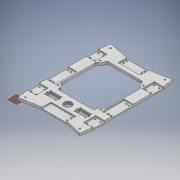
# Autodesk Inventor part: 3枚目
Saved by Autodesk Inventor 2018 (Build 220112000, 112)
## iProperties
Created: 2018-08-16
Part Number: 3枚目
Material: 一般
Document SubType Name: Modeling
Designer: shun2
Density: 1 g/cm^3
Appearance: 既定
Author: shun2
Autodesk Inventor part; units mm, degrees
ref_plane "YZ Plane" through (0, 0, 0) normal (1, 0, 0) x (0, 1, 0)
ref_plane "XZ Plane" through (0, 0, 0) normal (0, 1, 0) x (-1, 0, 0)
ref_plane "XY Plane" through (0, 0, 0) normal (0, 0, 1) x (1, 0, 0)
ref_plane "作業平面1" through (0, 0, 5.5) normal (0, 0, 1) x (1, 0, 0)
sketch "スケッチ3" plane through (0, 0, 5.5) normal (0, 0, 1) x (1, 0, 0)
  line L0 (0, 171.7239) -> (0, 23)
  line L1 (0, 23) -> (3, 0)
  line L2 (136, 23) -> (136, 171.7239)
  line L3 (136, 171.7239) -> (133.0079, 194.6636)
  line L4 (0, 23) -> (0, 75)
  line L5 (0, 127.7239) -> (0, 171.7239)
  line L6 (136, 171.7239) -> (136, 119.7239)
  line L7 (136, 67) -> (136, 23)
  circle A0 centre (11, 186.7239) radius 1.6
  circle A1 centre (125, 186.7239) radius 1.6
  circle A2 centre (11, 8) radius 1.6
  circle A3 centre (125, 8) radius 1.6
  line L8 (6.4, 186.7239) -> (15.6, 186.7239)
  line L9 (11, 182.1239) -> (11, 191.3239)
  line L10 (120.4, 186.7239) -> (129.6, 186.7239)
  line L11 (125, 182.1239) -> (125, 191.3239)
  line L12 (6.4, 8) -> (15.6, 8)
  line L13 (11, 3.4) -> (11, 12.6)
  line L14 (120.4, 8) -> (129.6, 8)
  line L15 (0, 127.7239) -> (0, 171.7239)
  line L16 (136, 171.7239) -> (136, 119.7239)
  line L17 (136, 67) -> (136, 23)
  line L18 (0, 23) -> (0, 75)
  line L19 (133, 0) -> (136, 23)
  line L20 (136, 46) -> (136, 23)
  line L21 (136, 23) -> (117.7, 23)
  line L22 (117.7, 23) -> (117.7, 48.5)
  line L23 (117.7, 48.5) -> (136, 48.5)
  line L24 (136, 48.5) -> (136, 23)
  line L25 (0, 23) -> (18.3, 23)
  line L26 (18.3, 23) -> (18.3, 48.5)
  line L27 (18.3, 48.5) -> (0, 48.5)
  line L28 (0, 48.5) -> (0, 23)
  line L29 (136, 171.7239) -> (117.7, 171.7239)
  line L30 (117.7, 171.7239) -> (117.7, 146.2239)
  line L31 (117.7, 146.2239) -> (136, 146.2239)
  line L32 (136, 146.2239) -> (136, 171.7239)
  line L33 (0, 171.7239) -> (18.3, 171.7239)
  line L34 (18.3, 171.7239) -> (18.3, 146.2239)
  line L35 (18.3, 146.2239) -> (0, 146.2239)
  line L36 (0, 146.2239) -> (0, 171.7239)
  circle A4 centre (132, 27) radius 1.6
  circle A5 centre (121.2, 27) radius 1.6
  circle A6 centre (132, 44.5) radius 1.6
  circle A7 centre (121.2, 44.5) radius 1.6
  circle A8 centre (132, 150.2239) radius 1.6
  circle A9 centre (132, 167.7239) radius 1.6
  circle A10 centre (121.2, 150.2239) radius 1.6
  circle A11 centre (121.2, 167.7239) radius 1.6
  circle A12 centre (14.8, 27) radius 1.6
  circle A13 centre (4, 27) radius 1.6
  circle A14 centre (14.8, 44.5) radius 1.6
  circle A15 centre (4, 44.5) radius 1.6
  circle A16 centre (14.8, 150.2239) radius 1.6
  circle A17 centre (4, 150.2239) radius 1.6
  circle A18 centre (14.8, 167.7239) radius 1.6
  circle A19 centre (4, 167.7239) radius 1.6
  line L37 (98, 8) -> (133, 0)
  line L38 (46.1667, 8) -> (3, 0)
  line L39 (98, 8) -> (46.1667, 8)
  line L40 (46.1667, 8) -> (46.1667, 26.3)
  line L41 (46.1667, 26.3) -> (98, 26.3)
  line L42 (98, 26.3) -> (98, 8)
  circle A20 centre (94, 12.65) radius 1.6
  circle A21 centre (94, 21.65) radius 1.6
  line L43 (68, 186.7239) -> (90.813, 186.7239)
  line L44 (90.813, 186.7239) -> (90.813, 168.4239)
  line L45 (90.813, 168.4239) -> (68, 168.4239)
  line L46 (133.0079, 194.6636) -> (90.813, 186.7239)
  line L47 (0, 171.7239) -> (2.9921, 194.6636)
  line L48 (68, 186.7239) -> (45.187, 186.7239)
  line L49 (45.187, 186.7239) -> (45.187, 168.4239)
  line L50 (45.187, 168.4239) -> (68, 168.4239)
  line L51 (2.9921, 194.6636) -> (45.187, 186.7239)
  circle A22 centre (86.313, 182.7239) radius 1.6
  circle A23 centre (48.5798, 182.7239) radius 1.6
  circle A24 centre (86.313, 176.7239) radius 1.6
  circle A25 centre (48.5798, 176.7239) radius 1.6
  point P0 (0, 0)
  point P1 (0, 179.7239)
  dimension "d134" = 18.3
  dimension "d137" = 3.2
  dimension "d139" = 3.2
  dimension "d196" = 22.813
  dimension "d197" = 18.3
  dimension "d198" = 3.2
  dimension "d199" = 4.5
  dimension "d200" = 4
  dimension "d201" = 3.2
  dimension "d202" = 3.2
  dimension "d203" = 10
  dimension "d204" = 3.2
  constraints: 104 end point, 26 centre point, 10 parallel, 6 horizontal, 6 perpendicular, 2 point on line
  measures "d134" distance of L39.end L40.end
  measures "d137" diameter of A20
  measures "d139" diameter of A21
  measures "d196" distance of L43.start L43.end
  measures "d197" distance of L43.end L44.end
  measures "d198" diameter of A22
  measures "d199" distance from line of A22.centre L44
  measures "d200" distance from line of L43 A22.centre
  measures "d201" diameter of A23
  measures "d202" diameter of A24
  measures "d203" distance from line of L43 A24.centre
  measures "d204" diameter of A25
ref_plane "作業平面6" through (0, 0, 5.5) normal (0, 0, 1) x (1, 0, 0)
ref_plane "作業平面7" through (0, 0, 5.5) normal (0, 0, -1) x (-1, 0, 0)
sketch "スケッチ9" plane through (0, 0, 5.5) normal (0, 0, -1) x (-1, 0, 0)
  line L0 (0, 146.2239) -> (0, 48.5)
  line L1 (0, 48.5) -> (0, 75)
  line L2 (0, 127.7239) -> (0, 146.2239)
  line L3 (0, 127.7239) -> (0, 146.2239)
  line L4 (0, 48.5) -> (0, 75)
  line L5 (-136, 171.7239) -> (-133.0079, 194.6636)
  circle A0 centre (-11, 186.7239) radius 1.6
  circle A1 centre (-125, 186.7239) radius 1.6
  circle A2 centre (-11, 8) radius 1.6
  circle A3 centre (-125, 8) radius 1.6
  line L6 (-6.4, 186.7239) -> (-15.6, 186.7239)
  line L7 (-11, 182.1239) -> (-11, 191.3239)
  line L8 (-120.4, 186.7239) -> (-129.6, 186.7239)
  line L9 (-125, 182.1239) -> (-125, 191.3239)
  line L10 (-6.4, 8) -> (-15.6, 8)
  line L11 (-11, 3.4) -> (-11, 12.6)
  line L12 (-120.4, 8) -> (-129.6, 8)
  line L13 (-133, 0) -> (-136, 23)
  line L14 (-136, 23) -> (-117.7, 23)
  line L15 (-117.7, 23) -> (-117.7, 48.5)
  line L16 (-117.7, 48.5) -> (-136, 48.5)
  line L17 (0, 23) -> (-18.3, 23)
  line L18 (-18.3, 23) -> (-18.3, 48.5)
  line L19 (-18.3, 48.5) -> (0, 48.5)
  line L20 (-117.7, 171.7239) -> (-117.7, 146.2239)
  line L21 (-117.7, 146.2239) -> (-136, 146.2239)
  circle A4 centre (-132, 27) radius 1.6
  circle A5 centre (-121.2, 27) radius 1.6
  circle A6 centre (-132, 44.5) radius 1.6
  circle A7 centre (-121.2, 44.5) radius 1.6
  circle A8 centre (-132, 150.2239) radius 1.6
  circle A9 centre (-132, 167.7239) radius 1.6
  circle A10 centre (-121.2, 150.2239) radius 1.6
  circle A11 centre (-121.2, 167.7239) radius 1.6
  circle A12 centre (-14.8, 27) radius 1.6
  circle A13 centre (-4, 27) radius 1.6
  circle A14 centre (-14.8, 44.5) radius 1.6
  circle A15 centre (-4, 44.5) radius 1.6
  line L22 (-98, 8) -> (-133, 0)
  line L23 (-46.1667, 8) -> (-3, 0)
  line L24 (-46.1667, 26.3) -> (-98, 26.3)
  line L25 (-98, 26.3) -> (-98, 8)
  circle A16 centre (-94, 12.65) radius 1.6
  circle A17 centre (-94, 21.65) radius 1.6
  circle A18 centre (-4, 150.2239) radius 1.6
  circle A19 centre (-14.8, 150.2239) radius 1.6
  circle A20 centre (-4, 167.7239) radius 1.6
  circle A21 centre (-14.8, 167.7239) radius 1.6
  line L26 (0, 0) -> (0, 23) construction
  line L27 (-136, 171.7239) -> (-117.7, 171.7239) projected
  line L28 (-117.7, 171.7239) -> (-136, 171.7239)
  line L29 (0, 48.5) -> (0, 146.2239) construction
  line L30 (0, 171.7239) -> (0, 236.1886) construction
  line L31 (0, 171.7239) -> (-3, 194.7239)
  line L32 (-18.3, 146.2239) -> (0, 146.2239)
  line L33 (-18.3, 171.7239) -> (-18.3, 146.2239)
  line L34 (-18.3, 146.2239) -> (0, 146.2239)
  line L35 (-18.3, 171.7239) -> (0, 171.7239) projected
  line L36 (0, 171.7239) -> (-18.3, 171.7239)
  line L37 (-136, 48.5) -> (-136, 146.2239)
  line L38 (-46.1667, 8) -> (-46.1667, 26.3)
  line L39 (0, 23) -> (-18.3, 23) projected
  line L40 (-3, 0) -> (0, 23)
  line L41 (-133.0079, 194.6636) -> (-90.813, 186.7239) projected
  line L42 (-136, 171.7239) -> (-133.0079, 194.6636) projected
  line L43 (-68, 186.7239) -> (-90.813, 186.7239) projected
  line L44 (-90.813, 186.7239) -> (-90.813, 168.4239) projected
  circle A22 centre (-86.313, 182.7239) radius 1.6 projected
  circle A23 centre (-86.313, 176.7239) radius 1.6 projected
  line L45 (-90.813, 168.4239) -> (-68, 168.4239) projected
  line L46 (-45.187, 168.4239) -> (-68, 168.4239) projected
  line L47 (-45.187, 186.7239) -> (-45.187, 168.4239) projected
  circle A24 centre (-48.5798, 176.7239) radius 1.6 projected
  circle A25 centre (-48.5798, 182.7239) radius 1.6 projected
  line L48 (-68, 186.7239) -> (-45.187, 186.7239) projected
  line L49 (-2.9921, 194.6636) -> (-45.187, 186.7239) projected
  line L50 (0, 171.7239) -> (-2.9921, 194.6636) projected
  point P0 (0, 179.7239)
  point P1 (-90.1667, 186.7239)
  point P2 (-42, 173.0739)
  point P3 (-42, 182.0739)
  dimension "d150" = 3.2
  dimension "d151" = 3.2
  dimension "d152" = 3.2
  dimension "d153" = 3.2
  constraints: 76 end point, 22 centre point, 5 vertical, 1 collinear, 1 horizontal, 1 perpendicular, 1 point on line, 1 other
  measures "d150" diameter of A18
  measures "d151" diameter of A19
  measures "d152" diameter of A20
  measures "d153" diameter of A21
extrude "押し出し9" add sketch "スケッチ9" against normal blind 5.5 contours L0 L19 L18 L17 L40 L23 L38 L24 L25 L22 L13 L14 L15 L16 L37 L21 L20 L27 L5 L41 L44 L45 L46 L47 L49 L31 L35 L33 L32
ref_plane "作業平面8" through (0, 0, 5.5) normal (0, 0, -1) x (-1, 0, 0)
sketch "スケッチ10" plane through (0, 0, 5.5) normal (0, 0, -1) x (-1, 0, 0)
  line L0 (0, 0) -> (0, 225.6064) construction
  line L1 (-115.4771, 146.7917) -> (-115.4771, 70.7387)
  line L2 (-21.0466, 70.5814) -> (-21.0466, 146.949)
  circle A0 centre (-22.8441, 153.1633) radius 1.6
  arc A1 (-29.6711, 160.1936) -> (-21.0466, 146.949) centre (-18.3577, 158.1302) ccw
  line L3 (-29.6711, 160.1936) -> (-106.0844, 160.1936)
  circle A2 centre (-113.0141, 153.1633) radius 1.6
  arc A3 (-115.4771, 146.7917) -> (-106.0844, 160.1936) centre (-117.3977, 158.1302) ccw
  circle A4 centre (-113.0141, 64.2633) radius 1.6
  arc A5 (-106.2762, 56.4741) -> (-115.4771, 70.7387) centre (-117.3977, 59.4002) ccw
  line L4 (-106.2762, 56.4741) -> (-29.4792, 56.4741)
  circle A6 centre (-22.8441, 64.2633) radius 1.6
  arc A7 (-21.0466, 70.5814) -> (-29.4792, 56.4741) centre (-18.3577, 59.4002) ccw
  circle A8 centre (-68, 39.7463) radius 8
  circle A9 centre (-112.1992, 40.362) radius 1.15
  line L5 (-87.6992, 46.362) -> (-110.6992, 46.362)
  line L6 (-110.6992, 46.362) -> (-110.6992, 34.362)
  circle A10 centre (-86.1992, 40.362) radius 1.15
  line L7 (-110.6992, 34.362) -> (-87.6992, 34.362)
  line L8 (-87.6992, 34.362) -> (-87.6992, 46.362)
  circle A11 centre (-49.8008, 40.362) radius 1.15
  line L9 (-48.3008, 34.362) -> (-48.3008, 46.362)
  line L10 (-48.3008, 46.362) -> (-25.3008, 46.362)
  line L11 (-25.3008, 34.362) -> (-48.3008, 34.362)
  line L12 (-25.3008, 46.362) -> (-25.3008, 34.362)
  circle A12 centre (-23.8008, 40.362) radius 1.15
  point P0 (-117.7, 161.7899)
  point P1 (-18.0035, 58.8386)
  point P2 (-68, 87.4279)
  point P3 (-67.8777, 108.7652)
  constraints: 26 end point, 13 centre point, 8 point on circle, 1 vertical
extrude "押し出し10" cut sketch "スケッチ10" against normal blind 5.5
sketch "スケッチ13" plane through (0, 0, 11) normal (0, 0, 1) x (1, 0, 0)
  line L0 (117.7, 62.936) -> (117.7, 108.562)
  line L1 (117.7, 62.936) -> (136, 62.936)
  line L2 (136, 108.562) -> (136, 62.936)
  line L3 (117.7, 108.562) -> (136, 108.562)
  line L4 (18.3, 108.562) -> (18.3, 62.936)
  line L5 (18.3, 108.562) -> (0, 108.562)
  line L6 (0, 62.936) -> (0, 108.562)
  line L7 (18.3, 62.936) -> (0, 62.936)
  line L8 (136, 48.5) -> (136, 146.2239) projected
  line L9 (136, 58.9751) -> (136, 64.08)
  point P0 (120.6031, 62.936)
  point P1 (244.1196, 130.8174)
  point P2 (0, 62.936)
  point P3 (15.3969, 108.562)
  dimension "d207" = 45.626
  dimension "d212" = 0
  dimension "d226" = 18.3
  constraints: 18 end point, 4 point on line
  measures "d207" distance between parallel lines of L3 L1
  measures "d212" distance between parallel lines of L2 L8
  measures "d226" distance between parallel lines of L0 L8
extrude "押し出し13" cut sketch "スケッチ13" against normal blind 2.5
sketch "スケッチ14" plane through (132, 67.436, 11) normal (0, 0, 1) x (1, 0, 0)
  circle A0 centre (-128, 36.626) radius 1.6
  circle A1 centre (-122, 36.626) radius 1.6
  circle A2 centre (-128, 0) radius 1.6
  circle A3 centre (-122, 0) radius 1.6
  circle A4 centre (-6, 36.626) radius 1.6
  circle A5 centre (0, 36.626) radius 1.6
  circle A6 centre (-6, 0) radius 1.6
  circle A7 centre (0, 0) radius 1.6
  circle A8 centre (-6, 0) radius 1.6423 projected
  point P0 (-132.5, -84.3342)
  constraints: 8 centre point, 7 coincident
extrude "押し出し14" cut sketch "スケッチ14" against normal blind 5.5 contours A0 | A1 | A2 | A3 | A4 | A5 | A6 | A7
extrude "押し出し15" add sketch "スケッチ3" along normal blind 2.7 contours L33 L34 L35 L0 | L48 L43 L44 L45 L50 L49 | L27 L26 L25 L0 | L2 L31 L30 L29 | L40 L41 L42 L39 | L21 L22 L23 L2
fillet "フィレット1" radius 3 8 edges at (29.6711, 160.1936, 8.25) (21.0466, 146.949, 8.25) (21.0466, 70.5814, 8.25) (29.4792, 56.4741, 8.25) (115.4771, 70.7387, 8.25) (106.2762, 56.4741, 8.25) (106.0844, 160.1936, 8.25) (115.4771, 146.7917, 8.25)
sketch "スケッチ15" plane through (0, 0, 11) normal (0, 0, 1) x (1, 0, 0)
  line L0 (25.3008, 46.362) -> (25.3008, 34.362) projected
  circle A0 centre (25.3008, 34.362) radius 1
  circle A1 centre (25.3008, 46.362) radius 1
  line L1 (48.3008, 46.362) -> (48.3008, 34.362) projected
  circle A2 centre (48.3008, 34.362) radius 1
  circle A3 centre (48.3008, 46.362) radius 1
  line L2 (87.6992, 34.362) -> (87.6992, 46.362) projected
  circle A4 centre (87.6992, 46.362) radius 1
  circle A5 centre (87.6992, 34.362) radius 1
  line L3 (110.6992, 34.362) -> (87.6992, 34.362) projected
  circle A6 centre (110.6992, 34.362) radius 1
  circle A7 centre (110.6992, 46.362) radius 1
  point P0 (0, 0)
  dimension "d230" = 2
  dimension "d231" = 2
  dimension "d232" = 2
  dimension "d233" = 2
  dimension "d234" = 2
  dimension "d235" = 2
  dimension "d236" = 2
  dimension "d237" = 2
  constraints: 8 centre point, 3 coincident
  measures "d230" diameter of A0
  measures "d231" diameter of A1
  measures "d232" diameter of A2
  measures "d233" diameter of A3
  measures "d234" diameter of A4
  measures "d235" diameter of A5
  measures "d236" diameter of A6
  measures "d237" diameter of A7
extrude "押し出し16" cut sketch "スケッチ15" against normal blind 10
